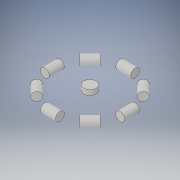
# Autodesk Inventor part: Ring
Saved by Autodesk Inventor 2019 (Build 230136000, 136)
## iProperties
Created: 2019-11-12
Part Number: Ring
Material: Generic
Document SubType Name: Modeling
Designer: Jorian Brusind
Density: 1 g/cm^3
Appearance: Default
Author: Jorian Brusind
Autodesk Inventor part; units mm, degrees
ref_plane "YZ Plane" through (0, 0, 0) normal (1, 0, 0) x (0, 1, 0)
ref_plane "XZ Plane" through (0, 0, 0) normal (0, 1, 0) x (-1, 0, 0)
ref_plane "XY Plane" through (0, 0, 0) normal (0, 0, 1) x (1, 0, 0)
sketch "Sketch4" plane through (0, 0, 0) normal (0, 0, 1) x (1, 0, 0)
  line L0 (0, 0) -> (15, 0)
  circle A0 centre (15, 0) radius 1.75
  dimension "d3" = 15
  dimension "d4" = 3.5
  constraints: 2 end point, 1 centre point, 1 coincident, 1 horizontal
  measures "d3" distance of L0.start L0.end
  measures "d4" diameter of A0
extrude "Extrusion1" add sketch "Sketch4" along normal mid plane 6
sketch "Sketch5" plane through (0, 0, 0) normal (0, 1, 0) x (-1, 0, 0)
  circle A0 centre (0, 0) radius 2.5
  dimension "d7" = 5
  constraints: 1 centre point, 1 coincident
  measures "d7" diameter of A0
extrude "Extrusion2" add sketch "Sketch5" along normal blind 2
pattern_circular "Circular Pattern1" count 8 over 360 about axis through (0, 0, 0) along (0, 1, 0) of "Extrusion1"
body "Solid4"
